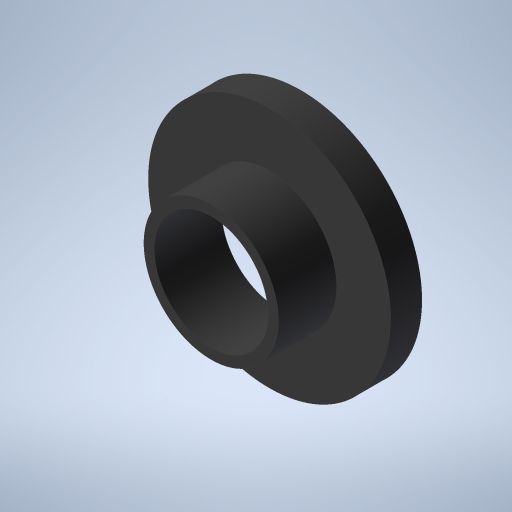
# Autodesk Inventor part: Part6
Saved by Autodesk Inventor 2024 (Build 280153000, 153)
## iProperties
Created: 2024-06-15
Part Number: Part6
Material: Generic
Document SubType Name: Sheet Metal
Designer: albah
Density: 1 g/cm^3
Sheet Metal Rule: Default_mm
Appearance: Default
Author: albah
Autodesk Inventor part; units mm, degrees
ref_plane "YZ Plane" through (0, 0, 0) normal (1, 0, 0) x (0, 1, 0)
ref_plane "XZ Plane" through (0, 0, 0) normal (0, 1, 0) x (-1, 0, 0)
ref_plane "XY Plane" through (0, 0, 0) normal (0, 0, 1) x (1, 0, 0)
sketch "Sketch1" plane through (0, 0, 0) normal (0, 0, 1) x (1, 0, 0)
  circle A0 centre (0, 0) radius 12.7
  circle A1 centre (0, 0) radius 15
  circle A2 centre (0, 0) radius 25.5
  circle A3 centre (0, 0) radius 27
  dimension "d1" = 25.4
  dimension "d2" = 30
  dimension "d3" = 51
  dimension "d4" = 54
  constraints: 4 centre point, 4 coincident
  measures "d1" diameter of A0
  measures "d2" diameter of A1
  measures "d3" diameter of A2
  measures "d4" diameter of A3
extrude "Extrusion1" add sketch "Sketch1" along normal blind 15 contours A1
extrude "Extrusion2" add sketch "Sketch1" along normal blind 2 contours A2
extrude "Extrusion3" add sketch "Sketch1" along normal blind 2 and the other way blind 5 contours A3
equation "\"BendRadius\" = Thickness"
equation "\"BendReliefWidth\" = Thickness"
equation "\"BendReliefDepth\" = 0.5 * Thickness"
equation "\"CornerReliefSize\" = 4 * Thickness"
equation "\"MinimumRemnant\" = 2 * Thickness"
equation "\"TransitionRadius\" = BendRadius"
equation "\"JacobiRadiusSize\" = BendRadius"
equation "\"GapSize\" = Thickness"
equation "\"Thickness\" = 0.5"
body "Solid1"
